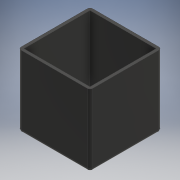
# Autodesk Inventor part: small_capsule
Saved by Autodesk Inventor 2017 (Build 210142000, 142)
## iProperties
Created: 2019-02-07
Part Number: small_capsule
Material: ABS Plastic
Document SubType Name: Modeling
Designer: felix
Density: 1.06 g/cm^3
Appearance: Smooth - Black
Author: felix
Autodesk Inventor part; units mm, degrees
ref_plane "YZ Plane" through (0, 0, 0) normal (1, 0, 0) x (0, 1, 0)
ref_plane "XZ Plane" through (0, 0, 0) normal (0, 1, 0) x (-1, 0, 0)
ref_plane "XY Plane" through (0, 0, 0) normal (0, 0, 1) x (1, 0, 0)
sketch "Sketch1" plane through (0, 0, 0) normal (0, 0, 1) x (1, 0, 0)
  line L0 (0, 0) -> (900, 0)
  line L1 (0, 0) -> (-900, 0)
  line L2 (0, 0) -> (0, -900)
  line L3 (0, 0) -> (0, 900)
  line L4 (-25, -25) -> (25, -25)
  line L5 (25, -25) -> (25, 25)
  line L6 (25, 25) -> (-25, 25)
  line L7 (-25, 25) -> (-25, -25)
  line L8 (-23, 23) -> (23, 23)
  line L9 (23, 23) -> (23, -23)
  line L10 (23, -23) -> (-23, -23)
  line L11 (-23, -23) -> (-23, 23)
  dimension "d0" = 900
  dimension "d1" = 900
  dimension "d2" = 900
  dimension "d3" = 900
  dimension "d4" = 25
  dimension "d5" = 25
  dimension "d6" = 25
  dimension "d7" = 25
  dimension "d9" = 2
  constraints: 24 end point, 4 parallel, 3 horizontal, 2 perpendicular, 2 vertical, 3 other
  measures "d0" distance of L0.start L0.end
  measures "d1" distance of L0.start L1.end
  measures "d2" distance of L0.start L2.end
  measures "d3" distance of L0.start L3.end
  measures "d4" distance between parallel lines of L3 L5
  measures "d5" distance between parallel lines of L0 L6
  measures "d6" distance between parallel lines of L2 L7
  measures "d7" distance between parallel lines of L0 L4
  measures "d9" distance between parallel lines of L6 L8
extrude "Extrusion1" add sketch "Sketch1" against normal blind 50
extrude "Extrusion2" cut sketch "Sketch1" against normal blind 48 contours L3 L8 L9 L0 | L2 L10 L11 L1 | L0 L9 L10 L2 | L1 L11 L8 L3
fillet "Fillet1" radius 2 8 edges at (-25, -25, -25) (-25, 25, -25) (25, 25, -25) (0, 25, -50) (25, -25, -25) (25, 0, -50) (0, -25, -50) (-25, 0, -50)
body "Solid1"
